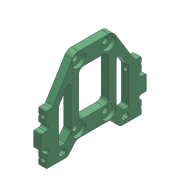
# Autodesk Inventor part: yaw_servo_side
Saved by Autodesk Inventor 2019.4 (Build 234330000, 330)
## iProperties
Created: 2018-08-06
Part Number: yaw_servo_side
Material: アルミニウム 6061
Document SubType Name: Modeling
Designer: student
Density: 2.7 g/cm^3
Appearance: 滑らか - 濃い海緑
Mass: 4.70379 g
Surface Area: 24.297 cm^2
Volume: 1.74214 cm^3
Author: student
Autodesk Inventor part; units mm, degrees
ref_plane "YZ Plane" through (0, 0, 0) normal (1, 0, 0) x (0, 1, 0)
ref_plane "XZ Plane" through (0, 0, 0) normal (0, 1, 0) x (-1, 0, 0)
ref_plane "XY Plane" through (0, 0, 0) normal (0, 0, 1) x (1, 0, 0)
sketch "スケッチ1" plane through (0, 0, 0) normal (1, 0, 0) x (0, 1, 0)
  line L0 (0, 0) -> (0, 38.5) construction
  circle A0 centre (6, 31.25) radius 1.3
  circle A1 centre (6, 7.25) radius 1.3
  line L1 (11.3843, 0) -> (19, 0)
  line L2 (19, 0) -> (19, 1.9)
  line L3 (19, 7) -> (21, 7)
  line L4 (21, 7) -> (21, 13)
  line L5 (21, 13) -> (19, 13)
  line L6 (19, 13) -> (19, 15) construction
  line L7 (19, 20) -> (17, 20)
  line L8 (16.1482, 20.4761) -> (8.5554, 32.8216)
  line L9 (6, 34.25) -> (0, 34.25)
  line L10 (0, 28.25) -> (4, 28.25)
  line L11 (6, 26.25) -> (6, 12.25)
  line L12 (4, 10.25) -> (0, 10.25)
  line L13 (13.8518, 19.4378) -> (10.8518, 24.3157)
  line L14 (9, 23.7918) -> (9, 8.7059)
  line L15 (14, 6) -> (14, 18.914)
  line L16 (21, 10) -> (17.9989, 10) construction
  line L17 (6, 31.25) -> (6, 7.25) construction
  line L18 (6, 19.25) -> (0, 19.25) construction
  arc A2 (6, 26.25) -> (4, 28.25) centre (4, 26.25) ccw
  arc A3 (4, 10.25) -> (6, 12.25) centre (4, 12.25) ccw
  line L19 (0, 4.25) -> (5.9529, 4.25)
  line L20 (7.485, 3.5356) -> (9.8522, 0.7144)
  arc A4 (10.8518, 24.3157) -> (9, 23.7918) centre (10, 23.7918) ccw
  arc A5 (14, 18.914) -> (13.8518, 19.4378) centre (13, 18.914) ccw
  arc A6 (7.485, 3.5356) -> (5.9529, 4.25) centre (5.9529, 2.25) ccw
  arc A7 (9.8522, 0.7144) -> (11.3843, 0) centre (11.3843, 2) ccw
  line L21 (6, 7.25) -> (0, 7.25) construction
  line L22 (6, 31.25) -> (0, 31.25) construction
  arc A8 (8.5554, 32.8216) -> (6, 34.25) centre (6, 31.25) ccw
  arc A9 (16.1482, 20.4761) -> (17, 20) centre (17, 21) ccw
  line L23 (6, 7.25) -> (9.9435, 2.5503) construction
  arc A10 (19, 18.1) -> (19, 16.9) centre (19.8, 17.5) ccw
  arc A11 (19, 3.1) -> (19, 1.9) centre (19.8, 2.5) ccw
  line L24 (19, 18.1) -> (19, 20)
  line L25 (19, 16.9) -> (19, 18.1) construction
  line L26 (19, 3.1) -> (19, 5)
  line L27 (19, 1.9) -> (19, 3.1) construction
  arc A12 (19, 15) -> (19, 13) centre (19, 14) ccw
  arc A13 (19, 7) -> (19, 5) centre (19, 6) ccw
  line L28 (19, 15) -> (19, 16.9)
  line L29 (19, 5) -> (19, 7) construction
  circle A14 centre (-6, 31.25) radius 1.3
  circle A15 centre (-6, 7.25) radius 1.3
  line L30 (-11.3843, 0) -> (-19, 0)
  line L31 (-19, 0) -> (-19, 1.9)
  line L32 (-19, 7) -> (-21, 7)
  line L33 (-21, 7) -> (-21, 13)
  line L34 (-21, 13) -> (-19, 13)
  line L35 (-19, 13) -> (-19, 15) construction
  line L36 (-19, 20) -> (-17, 20)
  line L37 (-16.1482, 20.4761) -> (-8.5554, 32.8216)
  line L38 (-6, 34.25) -> (0, 34.25)
  line L39 (0, 28.25) -> (-4, 28.25)
  line L40 (-6, 26.25) -> (-6, 12.25)
  line L41 (-4, 10.25) -> (0, 10.25)
  line L42 (-21, 10) -> (-17.9989, 10) construction
  arc A16 (-4, 28.25) -> (-6, 26.25) centre (-4, 26.25) ccw
  arc A17 (-6, 12.25) -> (-4, 10.25) centre (-4, 12.25) ccw
  line L43 (0, 4.25) -> (-5.9529, 4.25)
  line L44 (-7.485, 3.5356) -> (-9.8522, 0.7144)
  arc A18 (-5.9529, 4.25) -> (-7.485, 3.5356) centre (-5.9529, 2.25) ccw
  arc A19 (-11.3843, 0) -> (-9.8522, 0.7144) centre (-11.3843, 2) ccw
  arc A20 (-6, 34.25) -> (-8.5554, 32.8216) centre (-6, 31.25) ccw
  arc A21 (-17, 20) -> (-16.1482, 20.4761) centre (-17, 21) ccw
  arc A22 (-19, 16.9) -> (-19, 18.1) centre (-19.8, 17.5) ccw
  arc A23 (-19, 1.9) -> (-19, 3.1) centre (-19.8, 2.5) ccw
  line L45 (-19, 18.1) -> (-19, 20)
  line L46 (-19, 16.9) -> (-19, 18.1) construction
  line L47 (-19, 3.1) -> (-19, 5)
  line L48 (-19, 1.9) -> (-19, 3.1) construction
  arc A24 (-19, 13) -> (-19, 15) centre (-19, 14) ccw
  arc A25 (-19, 5) -> (-19, 7) centre (-19, 6) ccw
  line L49 (-19, 15) -> (-19, 16.9)
  line L50 (-19, 5) -> (-19, 7) construction
  line L51 (13, 3.6) -> (12, 3.6)
  line L52 (11, 2.6) -> (11, 2.4)
  line L53 (12, 1.4) -> (13, 1.4)
  line L54 (14, 2.4) -> (14, 2.6)
  arc A26 (14, 2.6) -> (13, 3.6) centre (13, 2.6) ccw
  arc A27 (13, 1.4) -> (14, 2.4) centre (13, 2.4) ccw
  arc A28 (11, 2.4) -> (12, 1.4) centre (12, 2.4) ccw
  arc A29 (12, 3.6) -> (11, 2.6) centre (12, 2.6) ccw
  line L55 (14, 2.5) -> (19.8, 2.5) construction
  line L56 (13, 5) -> (12.2705, 5)
  arc A30 (13, 5) -> (14, 6) centre (13, 6) ccw
  line L57 (11.5045, 5.3572) -> (9.234, 8.0631)
  arc A31 (11.5045, 5.3572) -> (12.2705, 5) centre (12.2705, 6) ccw
  arc A32 (9, 8.7059) -> (9.234, 8.0631) centre (10, 8.7059) ccw
  line L58 (-13.8518, 19.4378) -> (-10.8518, 24.3157)
  line L59 (-9, 23.7918) -> (-9, 8.7059)
  line L60 (-14, 6) -> (-14, 18.914)
  arc A33 (-9, 23.7918) -> (-10.8518, 24.3157) centre (-10, 23.7918) ccw
  arc A34 (-13.8518, 19.4378) -> (-14, 18.914) centre (-13, 18.914) ccw
  line L61 (-13, 3.6) -> (-12, 3.6)
  line L62 (-11, 2.6) -> (-11, 2.4)
  line L63 (-12, 1.4) -> (-13, 1.4)
  line L64 (-14, 2.4) -> (-14, 2.6)
  arc A35 (-13, 3.6) -> (-14, 2.6) centre (-13, 2.6) ccw
  arc A36 (-14, 2.4) -> (-13, 1.4) centre (-13, 2.4) ccw
  arc A37 (-12, 1.4) -> (-11, 2.4) centre (-12, 2.4) ccw
  arc A38 (-11, 2.6) -> (-12, 3.6) centre (-12, 2.6) ccw
  line L65 (-13, 5) -> (-12.2705, 5)
  arc A39 (-14, 6) -> (-13, 5) centre (-13, 6) ccw
  line L66 (-11.5045, 5.3572) -> (-9.234, 8.0631)
  arc A40 (-12.2705, 5) -> (-11.5045, 5.3572) centre (-12.2705, 6) ccw
  arc A41 (-9.234, 8.0631) -> (-9, 8.7059) centre (-10, 8.7059) ccw
  point P0 (16.441, 20)
  point P1 (14, 8.3105)
  point P2 (9, 5.9834)
  point P3 (-16.441, 20)
  point P4 (-6, 19.25)
  point P5 (-14, 8.3105)
  point P6 (-9, 5.9834)
  point P7 (-9.9435, 2.5503)
  point P8 (-14, 2.5)
  dimension "d0" = 20
  dimension "d1" = 6
  dimension "d2" = 2
  dimension "d3" = 38
  dimension "d4" = 12
  dimension "d5" = 2.6
  dimension "d6" = 24
  dimension "d7" = 7.25
  dimension "d14" = 2
  dimension "d16" = 1
  dimension "d19" = 3
  dimension "d20" = 2.5
  dimension "d21" = 2
  dimension "d22" = 3
  dimension "d24" = 1
  dimension "d25" = 2
  dimension "d26" = 50
  dimension "d27" = 5
  dimension "d28" = 0.8
  dimension "d29" = 1
  dimension "d30" = 15
  dimension "d31" = 1
  dimension "d44" = 1
  dimension "d45" = 2.2
  dimension "d46" = 3
  dimension "d48" = 1
  dimension "d49" = 1
  dimension "d50" = 1.25
  dimension "d51" = 3
  constraints: 132 end point, 76 point on circle, 72 horizontal alignment, 42 centre point, 32 tangent, 31 equal radius, 20 perpendicular, 18 collinear, 12 horizontal, 9 parallel, 9 point on line, 3 midpoint, 2 vertical, 1 concentric, 1 symmetric about line, 15 other
  measures "d0" distance between parallel lines of L7 L1
  measures "d1" distance of L3.end L4.end
  measures "d2" distance between parallel lines of L4 L2
  measures "d5" diameter of A1
  measures "d6" distance of L17.start L17.end
  measures "d7" distance from line of L1 L17.end
  measures "d14" radius of A2
  measures "d16" radius of A4
  measures "d19" distance between parallel lines of L11 L14
  measures "d20" distance between parallel lines of L8 L13
  measures "d21" radius of A6
  measures "d22" radius of A8
  measures "d24" radius of A9
  measures "d25" distance of L7.start L7.end
  measures "d26" angle of L19 L20
  measures "d27" distance between parallel lines of L15 L6
  measures "d28" distance from line of L6 A10.centre
  measures "d29" radius of A10
  measures "d30" distance of L55.end A10.centre
  measures "d31" radius of A12
  measures "d44" radius of A26
  measures "d45" distance between parallel lines of L53 L51
  measures "d46" distance between parallel lines of L54 L52
  measures "d48" radius of A30
  measures "d49" radius of A31
  measures "d50" distance between parallel lines of L20 L23
  measures "d51" distance between parallel lines of L23 L57
extrude "押し出し1" add sketch "スケッチ1" along normal blind 3
sketch "スケッチ2" plane through (3, 0, 0) normal (1, 0, 0) x (0, 0, -1)
  circle A0 centre (-31.25, 6) radius 1.3 construction
  circle A1 centre (-7.25, 6) radius 1.3 construction
  line L0 (0, 0) -> (-37.6662, 0) construction
  circle A2 centre (-31.25, 6) radius 2.8
  circle A3 centre (-7.25, 6) radius 2.8
  circle A4 centre (-31.25, -6) radius 2.8
  circle A5 centre (-7.25, -6) radius 2.8
  dimension "d34" = 5.6
  constraints: 4 centre point, 2 coincident, 2 end point, 2 symmetric about line, 1 equal radius, 1 horizontal, 2 other
  measures "d34" diameter of A2
extrude "押し出し2" cut sketch "スケッチ2" against normal blind 1.5
chamfer "面取り1" distance 0.25 angle 45 8 edges at (1.5, 19, 20) (1.5, 21, 13) (1.5, 21, 7) (1.5, 19, 0) (1.5, -19, 20) (1.5, -21, 13) (1.5, -21, 7) (1.5, -19, 0)
sketch "スケッチ3" plane through (0, 19, 16.9) normal (0, 1, 0) x (1, 0, 0)
  line L0 (0, -1.2) -> (3, -1.2) construction
  line L1 (1.5, -1.2) -> (1.5, 0) construction
  line L2 (0, 0) -> (3, 0) construction
  line L3 (0, 13.8) -> (3, 13.8) construction
  line L4 (1.5, 13.8) -> (1.5, 15) construction
  line L5 (0, 15) -> (3, 15) construction
  circle A0 centre (1.5, -0.6) radius 0.8
  circle A1 centre (1.5, 14.4) radius 0.8
  point P0 (0, 16.9)
  dimension "d40" = 1.6
  constraints: 6 midpoint, 4 end point, 2 centre point, 1 equal radius
  measures "d40" diameter of A0
extrude "押し出し3" cut sketch "スケッチ3" against normal blind 6
mirror "ミラー1" about plane through (0, 0, 0) normal (0, 1, 0) of "押し出し3"
